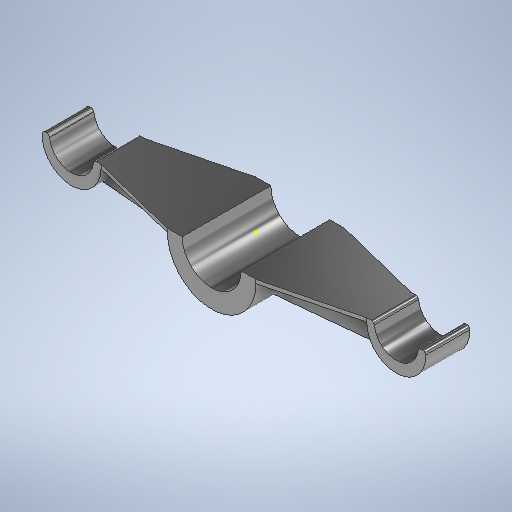
# Autodesk Inventor part: cad@58
Saved by Autodesk Inventor 2025.2 (Build 292293000, 293)
## iProperties
Created: 2025-04-10
Part Number: cad@58
Material: Generic
Document SubType Name: Modeling
Designer: spars
Density: 1 g/cm^3
Appearance: Chrome - Polished Black
Author: spars
Autodesk Inventor part; units mm, degrees
ref_plane "YZ Plane" through (0, 0, 0) normal (1, 0, 0) x (0, 1, 0)
ref_plane "XZ Plane" through (0, 0, 0) normal (0, 1, 0) x (-1, 0, 0)
ref_plane "XY Plane" through (0, 0, 0) normal (0, 0, 1) x (1, 0, 0)
sketch "Sketch1" plane through (0, 0, 0) normal (0, 0, 1) x (1, 0, 0)
  line L0 (-307.7131, 73.185043) -> (-155.934936, 73.185043) construction
  line L1 (-155.934936, 73.185043) -> (-155.934936, -78.169747) construction
  line L2 (-155.934936, -78.169747) -> (-307.7131, -78.169747) construction
  line L3 (-307.7131, -78.169747) -> (-307.7131, 73.185043) construction
  arc A0 (-30, 0) -> (30, 0) centre (0, 0) ccw
  arc A1 (-20, 2.5) -> (20, 2.5) centre (0, 2.5) ccw
  line L4 (20, 2.5) -> (30, 2.5)
  line L5 (-30, 0) -> (-30, 2.5)
  line L6 (30, 0) -> (30, 2.5)
  line L7 (-30, 2.5) -> (-20, 2.5)
  dimension "d4" = 30
  dimension "d7" = 20
  constraints: 8 end point, 4 point on circle, 2 centre point, 2 perpendicular, 2 other
  measures "d4" radius of A0
  measures "d7" radius of A1
extrude "Extrusion1" add sketch "Sketch1" along normal mid plane 60
sketch "Sketch2" plane through (0, 0, 0) normal (0, 1, 0) x (-1, 0, 0)
  point P0 (0, 0)
sketch "Sketch3" plane through (0, 0, 0) normal (0, 1, 0) x (-1, 0, 0)
  point P0 (0, 0)
sketch "Sketch4" plane through (0, 0, 0) normal (0, 0, 1) x (1, 0, 0)
  point P0 (0, 0)
sketch "Sketch5" plane through (0, 0, 0) normal (0, 1, 0) x (-1, 0, 0)
  line L0 (30, -30) -> (30, 30) projected
  line L1 (90, -15) -> (30, -30)
  line L2 (90, 15) -> (30, 30)
  line L3 (30, -30) -> (30, 30)
  line L4 (90, -15) -> (90, 15)
  point P0 (0, 0)
  constraints: 8 end point, 1 collinear
extrude "Extrusion2" add sketch "Sketch5" along normal blind 2.5
sketch "Sketch6" plane through (0, 0, 0) normal (0, 0, 1) x (1, 0, 0)
  arc A0 (-129.992282, 0.555556) -> (-90, 0) centre (-110, 0) ccw
  line L0 (-93.118057, 2.5) -> (-90.156865, 2.5)
  arc A1 (-124.895832, 0.735294) -> (-95.104168, 0.735294) centre (-110, 2.5) ccw
  line L1 (-126.881943, 2.5) -> (-127.993054, 2.5)
  line L2 (-30, 2.5) -> (-90, 2.5)
  line L3 (-90.156865, 2.5) -> (-90, 2.5)
  line L4 (-90, 0) -> (-90, 2.5)
  line L5 (-90, 2.5) -> (-90, 0)
  arc A2 (-93.118057, 2.5) -> (-95.104168, 0.735294) centre (-93.118057, 0.5) ccw
  arc A3 (-124.895832, 0.735294) -> (-126.881943, 2.5) centre (-126.881943, 0.5) ccw
  arc A4 (-127.993054, 2.5) -> (-129.992282, 0.555556) centre (-127.993054, 0.5) ccw
  point P0 (0, 0)
  point P1 (-129.843135, 2.5)
  point P2 (-95, 2.5)
  point P3 (-125, 2.5)
  dimension "d18" = 20
  dimension "d20" = 15
  dimension "d21" = 2
  constraints: 13 point on circle, 8 end point, 7 tangent, 5 centre point, 4 point on line, 2 equal radius, 2 horizontal, 1 perpendicular
  measures "d18" radius of A0
  measures "d20" radius of A1
  measures "d21" radius of A2
extrude "Extrusion3" add sketch "Sketch6" along normal mid plane 30
mirror "Mirror1" about plane through (0, 0, 0) normal (1, 0, 0) of "Extrusion2", "Extrusion3"
sketch "Sketch7" plane through (0, 0, 0) normal (0, 0, 1) x (1, 0, 0)
  arc A0 (-129.992282, 0.555556) -> (-90, 0) centre (-110, 0) ccw
  arc A1 (-129.992282, 0.555556) -> (-90, 0) centre (-110, 0) ccw
  arc A2 (-30, 0) -> (30, 0) centre (0, 0) ccw
  line L0 (-74.120165, -23.358526) -> (-36.738671, -26.770974)
  constraints: 2 end point
extrude "Rib1" add sketch "Sketch7" along normal mid plane 2.5 rib yes fills toward (-55.424872, -25.014957) open curves L0
mirror "Mirror2" about plane through (0, 0, 0) normal (1, 0, 0) of "Rib1"
body "Solid1"
